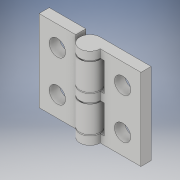
# Autodesk Inventor part: 26 scharnier 0.2 mm speling
Saved by Autodesk Inventor 2019 (Build 230136000, 136)
## iProperties
Created: 2021-01-06
Part Number: 26 scharnier 0.2 mm speling
Material: Generic
Document SubType Name: Modeling
Designer: semboonen
Density: 1 g/cm^3
Appearance: Default
Author: semboonen
Autodesk Inventor part; units mm, degrees
ref_plane "YZ Plane" through (0, 0, 0) normal (1, 0, 0) x (0, 1, 0)
sketch "Sketch1" plane through (0, 0, 0) normal (0, 0, 1) x (1, 0, 0)
  line L0 (12.5, -10) -> (12.5, 10)
  line L1 (-12.5, 10) -> (-12.5, -10)
  line L2 (-12.5, -10) -> (12.5, 10) construction
  line L3 (12.5, -10) -> (-12.5, 10) construction
  line L4 (2.5, -10) -> (2.5, 10)
  line L5 (-2.5, 10) -> (-2.5, -10)
  line L6 (-2.5, -10) -> (2.5, 10) construction
  line L7 (2.5, -10) -> (-2.5, 10) construction
  line L8 (12.5, 10) -> (2.5, 10)
  line L9 (-2.5, 10) -> (-12.5, 10)
  line L10 (-12.5, -10) -> (-2.5, -10)
  line L11 (2.5, -10) -> (12.5, -10)
  point P0 (0, 0)
  dimension "d0" = 25
  dimension "d1" = 20
  dimension "d2" = 5
  dimension "d3" = 20
  dimension "d4" = 38.66
  dimension "d5" = 75.964
  constraints: 24 end point, 4 equal length, 4 midpoint, 1 horizontal, 1 vertical
  measures "d0" distance of L1.start L0.end
  measures "d1" distance of L0.start L0.end
  measures "d2" distance of L5.start L4.end
  measures "d3" distance of L4.end L4.start
  measures "d4" angle of L8 L3
  measures "d5" angle of L11 L6
extrude "Extrusion1" add sketch "Sketch1" along normal blind 2.5
sketch "Sketch2" plane through (0, 0, 2.5) normal (0, 0, 1) x (1, 0, 0)
  line L0 (-2.5, -10) -> (-2.5, 10) projected
  line L1 (12.5, 10) -> (2.5, 10) projected
  line L2 (-2.5, 10) -> (0, 10)
  line L3 (2.5, 10) -> (2.5, -10) projected
  line L4 (-2.5, 10) -> (-2.5, 8)
  line L5 (-2.5, 8) -> (0, 5.5)
  line L6 (0, 5.5) -> (0, 10)
  line L7 (-2.5, 7.75) -> (0, 5.25)
  line L8 (-2.5, 7.75) -> (1.5, 7.75) construction
  line L9 (-2.5, 0) -> (-2.5, 1)
  line L10 (-2.5, 1) -> (0, 3.5)
  line L11 (0, 0) -> (0, 3.5)
  line L12 (-2.5, 1) -> (-2.5, 1.25) construction
  line L13 (-2.5, 1.25) -> (0, 3.75)
  line L14 (0, 3.75) -> (0, 5.25)
  line L15 (-2.5, 1.25) -> (-2.5, 7.75)
  line L16 (-2.5, -10) -> (0, -10)
  line L17 (-2.5, -10) -> (-2.5, -8)
  line L18 (-2.5, -8) -> (0, -5.5)
  line L19 (0, -5.5) -> (0, -10)
  line L20 (-2.5, -7.75) -> (0, -5.25)
  line L21 (-2.5, 0) -> (-2.5, -1)
  line L22 (-2.5, -1) -> (0, -3.5)
  line L23 (0, 0) -> (0, -3.5)
  line L24 (-2.5, -1) -> (-2.5, -1.25) construction
  line L25 (-2.5, -1.25) -> (0, -3.75)
  line L26 (0, -3.75) -> (0, -5.25)
  line L27 (-2.5, -1.25) -> (-2.5, -7.75)
  dimension "d11" = 2
  dimension "d12" = 135
  dimension "d14" = 45
  dimension "d15" = 1
  dimension "d17" = 135
  dimension "d18" = 0.25
  dimension "d19" = 90
  dimension "d20" = 90
  dimension "d21" = 90
  dimension "d22" = 90
  dimension "d23" = 90
  dimension "d24" = 90
  dimension "d25" = 90
  dimension "d26" = 2.5
  dimension "d27" = 2.25
  dimension "d28" = 2.5
  dimension "d29" = 6.1872
  dimension "d30" = 6.364
  dimension "d31" = 6.1872
  dimension "d32" = 6.364
  dimension "d33" = 12.5
  dimension "d34" = 12.5
  dimension "d35" = 1
  constraints: 50 end point, 8 parallel, 4 point on line, 2 horizontal, 1 collinear, 1 midpoint, 1 vertical
  measures "d11" distance of L0.end L4.end
  measures "d12" angle of L5 L4
  measures "d14" angle of L7 L8
  measures "d15" distance of L9.start L9.end
  measures "d17" angle of L9 L10
  measures "d18" distance of L9.end L12.end
  measures "d19" angle of L1 L11
  measures "d20" angle of L1 L23
  measures "d21" angle of L1 L26
  measures "d22" angle of L1 L21
  measures "d23" angle of L1 L24
  measures "d24" angle of L1 L27
  measures "d25" angle of L6 L1
  measures "d26" distance between parallel lines of L3 L14
  measures "d27" distance between parallel lines of L8 L1
  measures "d28" distance between parallel lines of L19 L3
  measures "d29" distance between parallel lines of L22 L7
  measures "d30" distance between parallel lines of L25 L7
  measures "d31" distance between parallel lines of L10 L20
  measures "d32" distance between parallel lines of L18 L10
  measures "d33" distance from line of L1.start L6
  measures "d34" distance from line of L1.start L26
  measures "d35" distance from line of L8.end L3
revolve "Revolution1" add sketch "Sketch2" angle 360 about axis through (0, 0, 2.5) along (0, 1, 0)
sketch "Sketch4" plane through (0, 0, 2.5) normal (0, 0, 1) x (1, 0, 0)
  line L0 (-2.5, -8) -> (-2.5, 8) projected
  line L1 (-2.5, 7.75) -> (-3.5, 7.75)
  line L2 (-3.5, 7.75) -> (-3.5, 10)
  line L3 (-3.5, 10) -> (-2.5, 10)
  line L4 (-2.5, 10) -> (-2.5, 7.75)
  line L5 (2.5, 10) -> (2.5, 8) projected
  line L6 (2.5, 8) -> (3.5, 8)
  line L7 (3.5, 8) -> (3.5, 1)
  line L8 (3.5, 1) -> (2.5, 1)
  line L9 (2.5, 1) -> (2.5, 8)
  line L10 (-2.5, -7.75) -> (-2.5, -1.25) projected
  line L11 (-2.5, -1.25) -> (-3.5, -1.25)
  line L12 (-3.5, -1.25) -> (-3.5, 1.25)
  line L13 (-3.5, 1.25) -> (-2.5, 1.25)
  line L14 (-2.5, 1.25) -> (-2.5, -1.25)
  line L15 (2.5, 1) -> (2.5, -1) projected
  line L16 (2.5, -1) -> (3.5, -1)
  line L17 (3.5, -1) -> (3.5, -8)
  line L18 (3.5, -8) -> (2.5, -8)
  line L19 (2.5, -8) -> (2.5, -1)
  line L20 (2.5, -7.75) -> (2.5, -7.75) projected
  line L21 (-2.5, -10) -> (-12.5, -10) projected
  line L22 (-2.5, -7.75) -> (-3.5, -7.75)
  line L23 (-3.5, -7.75) -> (-3.5, -10)
  line L24 (-3.5, -10) -> (-2.5, -10)
  line L25 (-2.5, -10) -> (-2.5, -7.75)
  point P0 (0, 0)
  dimension "d39" = 1
  dimension "d40" = 2.25
  dimension "d41" = 1
  dimension "d42" = 7
  dimension "d43" = 1
  dimension "d44" = 2.5
  dimension "d45" = 1
  dimension "d46" = 7
  dimension "d47" = 1
  constraints: 40 end point, 10 parallel, 5 horizontal, 5 perpendicular, 1 horizontal alignment, 1 point on line
  measures "d39" distance of L2.end L3.end
  measures "d40" distance of L1.end L2.end
  measures "d41" distance of L7.end L8.end
  measures "d42" distance of L6.end L7.end
  measures "d43" distance of L12.end L13.end
  measures "d44" distance of L11.end L12.end
  measures "d45" distance of L17.end L18.end
  measures "d46" distance of L16.end L17.end
  measures "d47" distance of L24.end L23.end
extrude "Extrusion3" cut sketch "Sketch4" against normal blind 2.5
sketch "Sketch5" plane through (0, 0, 2.5) normal (0, 0, 1) x (1, 0, 0)
  circle A0 centre (8, -5) radius 2
  line L0 (2.5, -10) -> (12.5, -10) projected
  line L1 (12.5, -10) -> (12.5, 10) projected
  line L2 (-12.5, 10) -> (-12.5, -10) projected
  line L3 (-12.5, -10) -> (-3.5, -10) projected
  circle A1 centre (8, 5) radius 2
  circle A2 centre (-8, -5) radius 2
  circle A3 centre (-8, 5) radius 2
  point P0 (0, 0)
  dimension "d50" = 4
  dimension "d51" = 5
  dimension "d52" = 4.5
  dimension "d57" = 10
  dimension "d60" = 16
  constraints: 4 centre point, 1 horizontal, 1 vertical, 6 other
  measures "d50" diameter of A0
  measures "d51" distance from line of L0 A0.centre
  measures "d52" distance from line of L1 A0.centre
  measures "d57" distance of A0.centre A1.centre
  measures "d60" distance of A0.centre A2.centre
extrude "Extrusion4" cut sketch "Sketch5" against normal blind 2.5
sketch "Sketch6" plane through (0, 0, 0) normal (0, 0, -1) x (-1, 0, 0)
  line L0 (2.5, 10) -> (-2.5, 10) projected
  line L1 (2.5, 8) -> (-2.5, 8) projected
  line L2 (-2.5, 10) -> (0, 10)
  line L3 (0, 10) -> (0, 8)
  line L4 (0, 8) -> (-2.5, 8)
  line L5 (-2.5, 8) -> (-2.5, 10)
  line L6 (2.5, -1) -> (-2.5, -1) projected
  line L7 (-2.5, 1) -> (0, 1)
  line L8 (0, 1) -> (0, -1)
  line L9 (0, -1) -> (-2.5, -1)
  line L10 (-2.5, -1) -> (-2.5, 1)
  line L11 (-2.5, -8) -> (-2.5, -10) projected
  line L12 (2.5, -10) -> (-2.5, -10) projected
  line L13 (-2.5, -8) -> (0, -8)
  line L14 (0, -8) -> (0, -10)
  line L15 (0, -10) -> (-2.5, -10)
  line L16 (-2.5, -10) -> (-2.5, -8)
  line L17 (2.5, -1.25) -> (0, -3.75) projected
  line L18 (0, -3.75) -> (2.5, -3.75)
  line L19 (2.5, -3.75) -> (2.5, -5.25)
  line L20 (2.5, -5.25) -> (0, -5.25)
  line L21 (0, -5.25) -> (0, -3.75)
  line L22 (2.5, 7.75) -> (0, 5.25) projected
  line L23 (0, 5.25) -> (2.5, 5.25)
  line L24 (2.5, 5.25) -> (2.5, 3.75)
  line L25 (2.5, 3.75) -> (0, 3.75)
  line L26 (0, 3.75) -> (0, 5.25)
  point P0 (0, 0)
  dimension "d65" = 5
  dimension "d66" = 6.25
  dimension "d67" = 15.25
  constraints: 40 end point, 10 parallel, 5 horizontal, 5 perpendicular, 5 point on line, 3 midpoint
  measures "d65" distance between parallel lines of L11 L19
  measures "d66" distance between parallel lines of L25 L0
  measures "d67" distance between parallel lines of L20 L0
extrude "Extrusion5" add sketch "Sketch6" against normal blind 2.5
ref_plane "Work Plane1" through (-2.5, -4.5, 0) normal (0, -1, 0) x (1, 0, 0)
sketch "Sketch7" plane through (-2.5, -4.5, 0) normal (0, -1, 0) x (1, 0, 0)
  line L0 (2.5, 0) -> (0, 0) projected
  line L1 (0, 0) -> (2.5, 0)
  line L2 (0, 0) -> (0, 2.5) projected
  line L3 (0, 0) -> (0, 2.5)
  line L4 (15, 0) -> (2.5, 0) projected
  arc A0 (0, 2.5) -> (2.5, 0) centre (2.5, 2.5) ccw
  constraints: 4 end point, 2 collinear, 2 point on circle, 1 centre point
extrude "Extrusion6" add sketch "Sketch7" along normal mid plane 6.5
ref_plane "Work Plane2" through (-2.5, 4.5, 0) normal (0, -1, 0) x (1, 0, 0)
sketch "Sketch8" plane through (-2.5, 4.5, 0) normal (0, -1, 0) x (1, 0, 0)
  arc A0 (0, 2.5) -> (2.5, 0) centre (2.5, 2.5) ccw projected
  line L0 (0, 2.5) -> (0, 0)
  line L1 (0, 0) -> (2.5, 0)
  line L2 (0, 2.5) -> (-1, 2.5) projected
  arc A1 (0, 2.5) -> (2.5, 0) centre (2.5, 2.5) ccw
  constraints: 4 end point, 2 point on circle, 2 tangent, 1 centre point, 1 concentric, 1 perpendicular, 1 vertical
extrude "Extrusion7" add sketch "Sketch8" along normal mid plane 6.5
body "Solid1"
